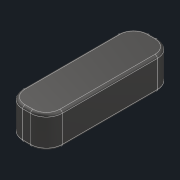
# Autodesk Inventor part: MCEN4000:G1K
Saved by Autodesk Inventor 2021 (Build 250183000, 183)
## iProperties
Created: 2020-10-21
Part Number: MCEN4000:G1K
Material: STEEL, AISI 1015
Document SubType Name: Modeling
Designer: Eugene Tang
Mass: 19.1409 g
Surface Area: 11.8955 cm^2
Volume: 2.43834 cm^3
Density: 7.85 g/cm^3
Appearance: Black Metal
Description: GEAR KEY (DIN 6885)
d0: 10.000 mm
d1: 8.000 mm
Author: Eugene Tang
Autodesk Inventor part; units mm, degrees
ref_plane "YZ Plane" through (0, 0, 0) normal (1, 0, 0) x (0, 1, 0)
ref_plane "XZ Plane" through (0, 0, 0) normal (0, 1, 0) x (-1, 0, 0)
ref_plane "XY Plane" through (0, 0, 0) normal (0, 0, 1) x (1, 0, 0)
sketch "Sketch1" plane through (0, 0, 0) normal (0, 0, 1) x (1, 0, 0)
  line L0 (-5, 4) -> (5, 4)
  line L1 (5, 4) -> (5, -4)
  line L2 (5, -4) -> (-5, -4)
  line L3 (-5, -4) -> (-5, 4)
  line L4 (-7, 0) -> (7, 0) construction
  line L5 (0, -5.6) -> (0, 5.6) construction
  point P0 (0, 0)
  point P1 (0, -4)
  point P2 (-5, 0)
  dimension "d0" = 10
  dimension "d1" = 8
  constraints: 8 end point, 2 midpoint, 2 parallel, 2 point on line, 1 horizontal, 1 perpendicular
  measures "d0" distance between parallel lines of L3 L1
  measures "d1" distance of L2.end L0.start
extrude "Extrusion1" add sketch "Sketch1" along normal blind 32
fillet "Fillet3" radius 4 4 edges at (5, 0, 32) (-5, 0, 32) (5, 0, 0) (-5, 0, 0)
fillet "Fillet1" radius 0.6 4 edges at (-5, 4, 16) (-5, -4, 16) (5, 4, 16) (5, -4, 16)
equation "\"d2\" = GearKey_L"
equation "\"TD\" = 0.45"
equation "\"Ball_DIA\" = 6"
equation "\"Screw_L\" = 292"
equation "\"Screw_DIA\" = 36"
equation "\"Nut_OD\" = 66"
equation "\"BPath_REVQ\" = 5.75"
equation "\"Tread_OFFSET\" = 8.075"
equation "\"SteeringColumn_DIA\" = 26"
equation "\"SteeringColumnChamfer_DEG\" = 20deg"
equation "\"Rack_L\" = 307.252"
equation "\"NutCapTread_L\" = 25"
equation "\"NutCapTread_THICKNESS\" = 5.365"
equation "\"SupportFlange_THICKNESS\" = 5"
equation "\"GearKey_L\" = 32"
body "Solid1"
